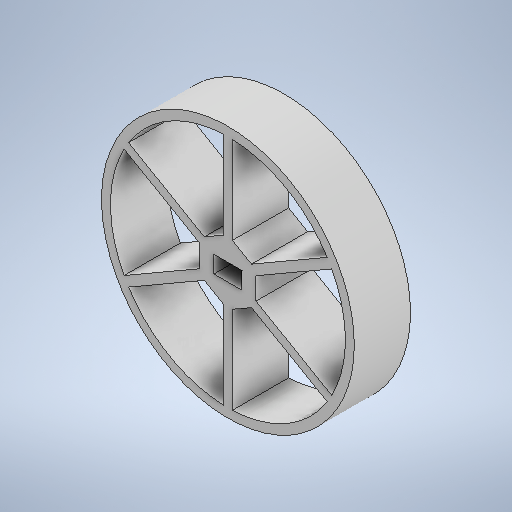
# Autodesk Inventor part: Wheel-D45B
Saved by Autodesk Inventor 2025.3 (Build 293356030, 356C)
## iProperties
Created: 2025-09-04
Part Number: Wheel-D45B
Material: 一般
Document SubType Name: Modeling
Designer: daisuke
Density: 1 g/cm^3
Appearance: 既定
Author: daisuke
Autodesk Inventor part; units mm, degrees
ref_plane "YZ Plane" through (0, 0, 0) normal (1, 0, 0) x (0, 1, 0)
ref_plane "XZ Plane" through (0, 0, 0) normal (0, 1, 0) x (-1, 0, 0)
ref_plane "XY Plane" through (0, 0, 0) normal (0, 0, 1) x (1, 0, 0)
sketch "スケッチ1" plane through (0, 0, 0) normal (0, 0, 1) x (1, 0, 0)
  line L0 (0, -5.7735) -> (-5, -2.8868)
  line L1 (-5, -2.8868) -> (-5, 2.8868)
  line L2 (-5, 2.8868) -> (0, 5.7735)
  line L3 (0, 5.7735) -> (5, 2.8868)
  line L4 (5, 2.8868) -> (5, -2.8868)
  line L5 (5, -2.8868) -> (0, -5.7735)
  circle A0 centre (0, 0) radius 22.5
  circle A1 centre (0, 0) radius 20.9
  dimension "HUB_D" = 10
  dimension "DIA" = 45
  dimension "RIM_THIN" = 1.6
  constraints: 12 end point, 3 coincident, 2 centre point, 1 vertical alignment, 13 other
  measures "HUB_D" distance between parallel lines of L4 L1
  measures "DIA" diameter of A0
  measures "RIM_THIN" radial gap between concentric circles of A0 A1
extrude "ハブ＆リム" add sketch "スケッチ1" along normal blind 10
sketch "スケッチ2" plane through (0, 0, 10) normal (0, 0, 1) x (1, 0, 0)
  line L0 (-0.8, 0) -> (0.8, 0)
  line L1 (0.8, 0) -> (0.8, 20.9)
  line L2 (0.8, 20.9) -> (-0.8, 20.9)
  line L3 (-0.8, 20.9) -> (-0.8, 0)
  line L4 (0, 0) -> (0, 25.5289) construction
  circle A0 centre (0, 0) radius 20.9 construction
  point P0 (0, 20.9)
  dimension "SPOKE_THIN" = 1.6
  constraints: 10 end point, 2 midpoint, 2 parallel, 1 horizontal, 1 perpendicular, 1 vertical, 1 vertical alignment, 1 other
  measures "SPOKE_THIN" distance between parallel lines of L1 L3
extrude "スポーク" add sketch "スケッチ2" against normal up to surface (10 mm away)
pattern_circular "円形状パターン1" count 6 over 360 about axis through (0, 0, -10) along (0, 0, 1) of "スポーク"
sketch "スケッチ3" plane through (0, 0, 10) normal (0, 0, 1) x (1, 0, 0)
  line L0 (-2.5, 1.525) -> (2.5, 1.525)
  line L1 (2.5, 1.525) -> (2.5, -1.525)
  line L2 (2.5, -1.525) -> (-2.5, -1.525)
  line L3 (-2.5, -1.525) -> (-2.5, 1.525)
  point P0 (0, 0)
  point P1 (0, 1.525)
  point P2 (2.5, 0)
  dimension "d11" = 5
  dimension "d12" = 3.05
  constraints: 8 end point, 2 midpoint, 2 parallel, 1 horizontal, 1 horizontal alignment, 1 perpendicular, 1 vertical alignment
  measures "d11" distance of L1.end L2.end
  measures "d12" distance of L0.end L1.end
extrude "押し出し3" cut sketch "スケッチ3" against normal through all
